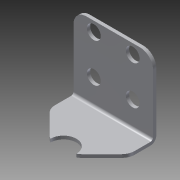
# Autodesk Inventor part: V5 Shooter Frame Channel Bracket (Guide Rail Version) P1
Saved by Autodesk Inventor 2014 SP1 (Build 180222100, 222)
## iProperties
Created: 2012-02-01
Part Number: V5 Shooter Frame Channel Bracket (Guide Rail Version) P1
Material: Aluminum-6061
Document SubType Name: Sheet Metal
Designer: Moses
Density: 2.71 g/cm^3
Sheet Metal Rule: Default
Mass: 8.62047 g
Surface Area: 44.3894 cm^2
Volume: 3.18099 cm^3
Flat Pattern Width: 3.89612 cm
Flat Pattern Length: 6.12228 cm
Flat Pattern Area: 23.8531 cm^2
Sheet Metal Width: 1.534 in
Sheet Metal Length: 2.410 in
Sheet Metal Area: 3.697 in^2
Appearance: Aluminum - Flat
Author: Moses
Autodesk Inventor part; units mm, degrees
ref_plane "YZ Plane" through (0, 0, 0) normal (1, 0, 0) x (0, 1, 0)
ref_plane "XZ Plane" through (0, 0, 0) normal (0, 1, 0) x (-1, 0, 0)
ref_plane "XY Plane" through (0, 0, 0) normal (0, 0, 1) x (1, 0, 0)
sketch "Sketch1" plane through (0, 0, 0) normal (0, 0, 1) x (1, 0, 0)
  line L0 (0, 0) -> (38.9612, 0)
  line L1 (38.9612, 0) -> (38.9612, 38.1)
  line L2 (38.9612, 38.1) -> (0, 38.1)
  line L3 (0, 38.1) -> (0, 0)
  line L4 (0, 0) -> (0, -38.1)
  line L5 (0, -38.1) -> (38.9612, -38.1)
  line L6 (38.9612, -38.1) -> (38.9612, 0)
  line L7 (0, -25.4) -> (38.9612, -25.4) construction
  circle A0 centre (29.0056, -25.4) radius 3.3782
  line L8 (-19.05, -25.4) -> (19.9112, -25.4) construction
  circle A1 centre (9.9556, -25.4) radius 3.3782
  line L9 (0, -6.35) -> (38.9612, -6.35) construction
  circle A2 centre (29.0056, -6.35) radius 3.3782
  line L10 (-19.05, -6.35) -> (19.9112, -6.35) construction
  circle A3 centre (9.9556, -6.35) radius 3.3782
  dimension "d0" = 38.9612
  dimension "d7" = 38.1
  dimension "d8" = 38.1
  dimension "d26" = 12.7
  dimension "d28" = 6.7564
  dimension "d30" = 9.9556
  dimension "d33" = 19.05
  dimension "d36" = 19.05
  constraints: 22 end point, 6 point on line, 4 centre point, 3 vertical, 2 horizontal, 2 parallel, 2 perpendicular, 15 other
  measures "d0" distance of L0.start L0.end
  measures "d7" distance between parallel lines of L0 L2
  measures "d8" distance of L0.start L4.end
  measures "d26" distance between parallel lines of L5 L7
  measures "d28" diameter of A0
  measures "d30" distance from line of L6 A0.centre
  measures "d33" distance of L7.start L8.start
  measures "d36" distance of L7.start L9.start
extrude "Plate1" add sketch "Sketch1" along normal blind 1.5875 contours L3 L2 L1 L0 | L0 L6 L5 L4 | A0 | A1 | A2 | A3
fold "Fold1" angle 90 bend radius 1.27 thickness 1.5875 k factor 0.44 line from (0, 0, 0) to (38.9612, 0, 0) line at bend end moving side (0, -1, 0) folds toward (0, 0, 1)
fillet "Corner Round1" radius 6.35 4 edges at (0, 38.1, 0.7937) (38.9612, 38.1, 0.7937) (38.9612, 1.0284, 40.9575) (0, 1.0284, 40.9575)
sketch "Sketch2" plane through (0, 0, 0) normal (0, 0, -1) x (-1, 0, 0)
  line L0 (-38.9612, 3.0921) -> (-38.9612, 31.75) projected
  line L1 (-38.9612, 3.0921) -> (0, 3.0921) projected
  line L2 (-32.6112, 38.1) -> (-6.35, 38.1) projected
  line L3 (0, 0.2346) -> (-38.9612, 0.2346) construction
  circle A0 centre (-29.0056, 33.2546) radius 3.3782
  circle A1 centre (-9.9556, 33.2546) radius 3.3782
  circle A2 centre (-29.0056, 14.2046) radius 3.3782
  circle A3 centre (-9.9556, 14.2046) radius 3.3782
  line L4 (-29.0056, 33.2546) -> (-9.9556, 33.2546) construction
  line L5 (-19.4806, 33.2546) -> (-19.4806, 3.0921) construction
  point P0 (0, 0)
  dimension "d42" = 19.05
  dimension "d45" = 19.05
  dimension "d48" = 6.7564
  dimension "d49" = 13.97
  constraints: 4 centre point, 4 end point, 2 midpoint, 2 vertical, 1 horizontal, 1 parallel, 6 other
  measures "d42" distance of L4.start L4.end
  measures "d45" distance of L4.start A2.centre
  measures "d48" diameter of A0
  measures "d49" distance from line of L3 A3.centre
extrude "Cut1" cut sketch "Sketch2" against normal blind 1.5875
sketch "Sketch3" plane through (0, 0.2346, 2.8575) normal (0, -1, 0) x (1, 0, 0)
  arc A0 (6.35, 38.1) -> (0, 31.75) centre (6.35, 31.75) ccw projected
  line L0 (0, 0) -> (0, 31.75) projected
  line L1 (38.9612, 31.75) -> (38.9612, 0) projected
  arc A1 (38.9612, 31.75) -> (32.6112, 38.1) centre (32.6112, 31.75) ccw projected
  line L2 (6.35, 38.1) -> (32.6112, 38.1) projected
  line L3 (38.9612, -2.8575) -> (0, -2.8575) construction
  circle A2 centre (19.4806, 23.1228) radius 6.35 projected
  line L4 (0, 23.1228) -> (38.9612, 23.1228) construction
  line L5 (0, 23.1228) -> (13.1306, 23.1228)
  line L6 (25.8306, 23.1228) -> (38.9612, 23.1228)
  constraints: 6 end point, 4 point on line, 2 point on circle, 1 collinear, 1 midpoint, 1 perpendicular
extrude "Extrusion1" cut sketch "Sketch3" against normal through all
chamfer "Corner Chamfer1" distance 12.7 angle 45 2 edges at (38.9612, 1.0284, 25.9803) (0, 1.0284, 25.9803)
fillet "Corner Round3" radius 6.35 4 edges at (38.9612, 1.0284, 13.2803) (0, 1.0284, 13.2803) (12.7, 1.0284, 25.9803) (26.2612, 1.0284, 25.9803)
equation "\"d0\" = p1channelwidth"
equation "\"d28\" = d3"
equation "\"d30\" = -0.5 * d22 + 0.5 * d0"
equation "\"d33\" = d22"
equation "\"d36\" = d22"
equation "\"d10\" = BendReliefWidth"
equation "\"d11\" = BendReliefDepth"
equation "\"d12\" = MinimumRemnant"
equation "\"d13\" = BendRadius"
equation "\"d42\" = p1holespacing"
equation "\"d45\" = p1holespacing"
equation "\"d48\" = p1mountholedia"
equation "\"d49\" = p1holedistedge"
equation "\"d50\" = Thickness"
equation "\"BendRadius\" = Thickness"
equation "\"BendReliefWidth\" = Thickness"
equation "\"BendReliefDepth\" = 0.5 * Thickness"
equation "\"CornerReliefSize\" = 4 * Thickness"
equation "\"MinimumRemnant\" = 2 * Thickness"
equation "\"TransitionRadius\" = BendRadius"
equation "\"JacobiRadiusSize\" = BendRadius"
equation "\"GapSize\" = Thickness"
equation "\"p1channelwidth\" = 38.96118"
equation "\"d3\" = d4"
equation "\"d4\" = p1mountholedia"
equation "\"d9\" = BendRadius"
equation "\"d22\" = p1holespacing"
equation "\"p1holespacing\" = 19.05"
equation "\"p1mountholedia\" = 6.7564"
equation "\"p1holedistedge\" = 13.97"
equation "\"Thickness\" = 1.5875"
body "Solid1"
